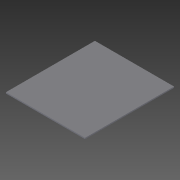
# Autodesk Inventor part: Base
Saved by Autodesk Inventor 2015 (Build 190159000, 159)
## iProperties
Created: 2014-08-22
Part Number: Base
Material: Generic
Document SubType Name: Modeling
Designer: t_clevj
Density: 1 g/cm^3
Appearance: Default
Author: t_clevj
Autodesk Inventor part; units mm, degrees
ref_plane "YZ Plane" through (0, 0, 0) normal (1, 0, 0) x (0, 1, 0)
ref_plane "XZ Plane" through (0, 0, 0) normal (0, 1, 0) x (-1, 0, 0)
ref_plane "XY Plane" through (0, 0, 0) normal (0, 0, 1) x (1, 0, 0)
sketch "Sketch1" plane through (0, 0, 0) normal (0, 0, 1) x (1, 0, 0)
  line L0 (380, -16) -> (-10, -16) projected
  line L1 (386, -16) -> (386, 456) projected
  line L2 (-10, 456) -> (380, 456) projected
  line L3 (386, 456) -> (-10, 456)
  line L4 (-10, 456) -> (-16, 456)
  line L5 (-16, 456) -> (-16, -16)
  line L6 (-16, -16) -> (-10, -16)
  line L7 (-10, -16) -> (386, -16)
  line L8 (386, -16) -> (386, 456)
  point P0 (0, 0)
  dimension "d0" = 6
  constraints: 12 end point, 3 collinear, 2 perpendicular, 1 point on line
  measures "d0" distance of L2.start L4.end
extrude "Extrusion1" add sketch "Sketch1" along normal blind 6
body "Solid1"
